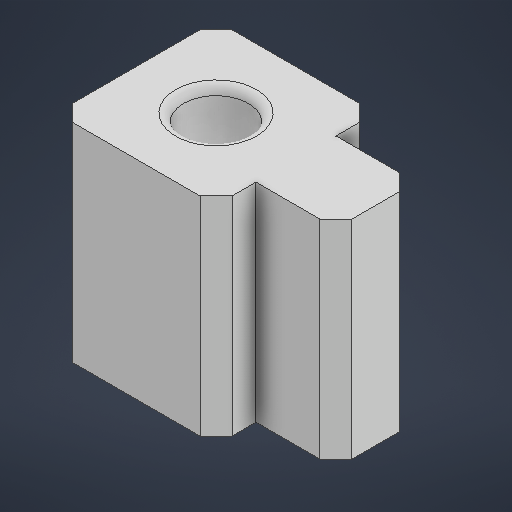
# Autodesk Inventor part: Turret_Holder_2
Saved by Autodesk Inventor 2026.2 (Build 302298000, 298)
## iProperties
Created: 2025-12-30
Part Number: Turret_Holder_2
Material: Generic
Document SubType Name: Modeling
Designer: Cobble
Density: 1 g/cm^3
Appearance: Default
Author: Cobble
Autodesk Inventor part; units mm, degrees
ref_plane "YZ Plane" through (0, 0, 0) normal (1, 0, 0) x (0, 1, 0)
ref_plane "XZ Plane" through (0, 0, 0) normal (0, 1, 0) x (-1, 0, 0)
ref_plane "XY Plane" through (0, 0, 0) normal (0, 0, 1) x (1, 0, 0)
sketch "Sketch1" plane through (0, 0, 0) normal (0, 0, 1) x (1, 0, 0)
  line L0 (0, 0) -> (20, 0)
  line L1 (20, 0) -> (20, 20)
  line L2 (20, 20) -> (0, 20)
  line L3 (0, 20) -> (0, 0)
  line L4 (-10, 5) -> (30, 5)
  line L5 (30, 5) -> (30, 15)
  line L6 (30, 15) -> (-10, 15)
  line L7 (-10, 15) -> (-10, 5)
  line L8 (-10, 5) -> (30, 15) construction
  line L9 (30, 5) -> (-10, 15) construction
  circle A0 centre (10, 10) radius 4.05
  point P0 (20, 5)
  point P1 (20, 15)
  dimension "d0" = 20
  dimension "d1" = 20
  dimension "d2" = 40
  dimension "d3" = 10
  dimension "d4" = 10
  dimension "d5" = 10
  dimension "d6" = 8.1
  constraints: 20 end point, 4 parallel, 2 horizontal, 2 midpoint, 2 perpendicular, 1 centre point, 1 coincident
  measures "d0" distance of L2.end L1.end
  measures "d1" distance of L1.end L0.end
  measures "d2" distance of L6.end L5.end
  measures "d3" distance of L5.end L4.end
  measures "d4" horizontal distance of point (10, 10) L2.end
  measures "d5" horizontal distance of point (10, 10) L2.end
  measures "d6" diameter of A0
extrude "Extrusion1" add sketch "Sketch1" along normal blind 26 contours L3 L4 L1 L0 | L3 L6 L1 L4 | L1 L6 L5 L4 | L3 L2 L1 L6
chamfer "Chamfer1" distance 2 angle 45 6 edges at (20, 20, 13) (30, 15, 13) (30, 5, 13) (20, 0, 13) (0, 20, 13) (0, 0, 13)
fillet "Fillet1" radius 1 2 edges at (5.95, 10, 0) (5.95, 10, 26)
body "Solid1"
